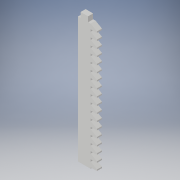
# Autodesk Inventor part: graduated_foot
Saved by Autodesk Inventor 2019.4 (Build 234330000, 330)
## iProperties
Created: 2019-12-14
Part Number: graduated_foot
Material: Generic
Document SubType Name: Modeling
Designer: fabfarm
Density: 1 g/cm^3
Appearance: Default
Author: fabfarm
Autodesk Inventor part; units mm, degrees
ref_plane "YZ Plane" through (0, 0, 0) normal (1, 0, 0) x (0, 1, 0)
ref_plane "XZ Plane" through (0, 0, 0) normal (0, 1, 0) x (-1, 0, 0)
ref_plane "XY Plane" through (0, 0, 0) normal (0, 0, 1) x (1, 0, 0)
sketch "Sketch4" plane through (0, 0, 0) normal (0, 0, 1) x (1, 0, 0)
  line L0 (0, 500) -> (50, 500)
  line L1 (50, 500) -> (50, 0)
  line L2 (50, 0) -> (0, 0)
  line L3 (0, 0) -> (0, 500)
  dimension "d31" = 50
  dimension "d32" = 500
  constraints: 8 end point, 2 parallel, 2 point on line, 1 horizontal, 1 perpendicular
  measures "d31" distance of L0.start L0.end
  measures "d32" distance of L2.end L0.start
extrude "Extrusion1" add sketch "Sketch4" along normal blind 20.18
sketch "Sketch5" plane through (0, 0, 20.18) normal (0, 0, 1) x (1, 0, 0)
  line L0 (50, 500) -> (0, 500) projected
  line L1 (10, 500) -> (40, 500)
  line L2 (40, 500) -> (40, 520.18)
  line L3 (40, 520.18) -> (10, 520.18)
  line L4 (10, 520.18) -> (10, 500)
  line L5 (0, 500) -> (0, 0) projected
  line L6 (50, 0) -> (50, 500) projected
  dimension "d46" = 10
  dimension "d47" = 10
  dimension "d48" = 20.18
  constraints: 8 end point, 2 parallel, 1 horizontal, 1 perpendicular, 1 point on line
  measures "d46" distance between parallel lines of L5 L4
  measures "d47" distance between parallel lines of L6 L2
  measures "d48" distance of L3.end L1.start
extrude "Extrusion2" add sketch "Sketch5" against normal blind 20.18
sketch "Sketch6" plane through (0, 0, 20.18) normal (0, 0, 1) x (1, 0, 0)
  line L0 (50, 500) -> (75, 485.5662)
  line L1 (75, 485.5662) -> (75, 480.5662)
  line L2 (75, 480.5662) -> (50, 480.5662)
  line L3 (50, 500) -> (40, 500) projected
  line L4 (40, 500) -> (50, 500) projected
  line L5 (50, 500) -> (50, 480.5662)
  line L6 (50, 0) -> (50, 500) projected
  line L7 (50, 472) -> (75, 457.5662)
  line L8 (75, 457.5662) -> (75, 452.5662)
  line L9 (75, 452.5662) -> (50, 452.5662)
  line L10 (50, 472) -> (50, 452.5662)
  line L11 (50, 444) -> (75, 429.5662)
  line L12 (75, 429.5662) -> (75, 424.5662)
  line L13 (75, 424.5662) -> (50, 424.5662)
  line L14 (50, 444) -> (50, 424.5662)
  line L15 (50, 416) -> (75, 401.5662)
  line L16 (75, 401.5662) -> (75, 396.5662)
  line L17 (75, 396.5662) -> (50, 396.5662)
  line L18 (50, 416) -> (50, 396.5662)
  line L19 (50, 388) -> (75, 373.5662)
  line L20 (75, 373.5662) -> (75, 368.5662)
  line L21 (75, 368.5662) -> (50, 368.5662)
  line L22 (50, 388) -> (50, 368.5662)
  line L23 (50, 360) -> (75, 345.5662)
  line L24 (75, 345.5662) -> (75, 340.5662)
  line L25 (75, 340.5662) -> (50, 340.5662)
  line L26 (50, 360) -> (50, 340.5662)
  line L27 (50, 332) -> (75, 317.5662)
  line L28 (75, 317.5662) -> (75, 312.5662)
  line L29 (75, 312.5662) -> (50, 312.5662)
  line L30 (50, 332) -> (50, 312.5662)
  line L31 (50, 304) -> (75, 289.5662)
  line L32 (75, 289.5662) -> (75, 284.5662)
  line L33 (75, 284.5662) -> (50, 284.5662)
  line L34 (50, 304) -> (50, 284.5662)
  line L35 (50, 276) -> (75, 261.5662)
  line L36 (75, 261.5662) -> (75, 256.5662)
  line L37 (75, 256.5662) -> (50, 256.5662)
  line L38 (50, 276) -> (50, 256.5662)
  line L39 (50, 248) -> (75, 233.5662)
  line L40 (75, 233.5662) -> (75, 228.5662)
  line L41 (75, 228.5662) -> (50, 228.5662)
  line L42 (50, 248) -> (50, 228.5662)
  line L43 (50, 220) -> (75, 205.5662)
  line L44 (75, 205.5662) -> (75, 200.5662)
  line L45 (75, 200.5662) -> (50, 200.5662)
  line L46 (50, 220) -> (50, 200.5662)
  line L47 (50, 192) -> (75, 177.5662)
  line L48 (75, 177.5662) -> (75, 172.5662)
  line L49 (75, 172.5662) -> (50, 172.5662)
  line L50 (50, 192) -> (50, 172.5662)
  line L51 (50, 164) -> (75, 149.5662)
  line L52 (75, 149.5662) -> (75, 144.5662)
  line L53 (75, 144.5662) -> (50, 144.5662)
  line L54 (50, 164) -> (50, 144.5662)
  line L55 (50, 136) -> (75, 121.5662)
  line L56 (75, 121.5662) -> (75, 116.5662)
  line L57 (75, 116.5662) -> (50, 116.5662)
  line L58 (50, 136) -> (50, 116.5662)
  line L59 (50, 108) -> (75, 93.5662)
  line L60 (75, 93.5662) -> (75, 88.5662)
  line L61 (75, 88.5662) -> (50, 88.5662)
  line L62 (50, 108) -> (50, 88.5662)
  line L63 (50, 80) -> (75, 65.5662)
  line L64 (75, 65.5662) -> (75, 60.5662)
  line L65 (75, 60.5662) -> (50, 60.5662)
  line L66 (50, 80) -> (50, 60.5662)
  line L67 (50, 52) -> (75, 37.5662)
  line L68 (75, 37.5662) -> (75, 32.5662)
  line L69 (75, 32.5662) -> (50, 32.5662)
  line L70 (50, 52) -> (50, 32.5662)
  line L71 (50, 24) -> (75, 9.5662)
  line L72 (75, 9.5662) -> (75, 4.5662)
  line L73 (75, 4.5662) -> (50, 4.5662)
  line L74 (50, 24) -> (50, 4.5662)
  point P0 (0, 0)
  point P1 (40, 472)
  point P2 (40, 444)
  point P3 (40, 416)
  point P4 (40, 388)
  point P5 (40, 360)
  point P6 (40, 332)
  point P7 (40, 304)
  point P8 (40, 276)
  point P9 (40, 248)
  point P10 (40, 220)
  point P11 (40, 192)
  point P12 (40, 164)
  point P13 (40, 136)
  point P14 (40, 108)
  point P15 (40, 80)
  point P16 (40, 52)
  point P17 (40, 24)
  dimension "d49" = 25
  dimension "d50" = 30
  dimension "d51" = 5
  dimension "d54" = 28
  constraints: 144 end point, 1 collinear, 1 horizontal, 1 perpendicular, 1 vertical, 153 other
  measures "d49" distance of L1.end L2.end
  measures "d50" angle of L3 L0
  measures "d51" distance of L0.end L1.end
  measures "d54" distance of L0.start L7.start
extrude "Extrusion3" add sketch "Sketch6" against normal blind 20.18
body "Solid1"
